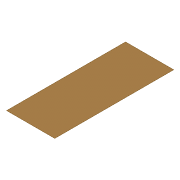
# Autodesk Inventor part: FE-00035-06
Saved by Autodesk Inventor 2012 (Build 160160000, 160)
## iProperties
Created: 2008-06-08
Part Number: FE-00035-06
Document SubType Name: Modeling
Designer: dfoster
Density: 1 g/cm^3
Description: Carpet, Playing Field
Material: Default
Title: Carpet, Playing Field
Author: dfoster
Autodesk Inventor part; units mm, degrees
ref_plane "YZ Plane" through (0, 0, 0) normal (1, 0, 0) x (0, 1, 0)
ref_plane "XZ Plane" through (0, 0, 0) normal (0, 1, 0) x (-1, 0, 0)
ref_plane "XY Plane" through (0, 0, 0) normal (0, 0, 1) x (1, 0, 0)
sketch "Sketch2" plane through (0, 0, 0) normal (0, 1, 0) x (-1, 0, 0)
  line L0 (4572, 11277.6) -> (-4572, 11277.6)
  line L1 (-4572, 11277.6) -> (-4572, -11277.6)
  line L2 (-4572, -11277.6) -> (4572, -11277.6)
  line L3 (4572, -11277.6) -> (4572, 11277.6)
  line L4 (0, -15788.64) -> (0, 15788.64) projected
  line L5 (-6400.8, 0) -> (6400.8, 0) projected
  dimension "d0" = 22555.2
  dimension "d1" = 9144
  dimension "d4" = 11277.6
  dimension "d5" = 4572
  constraints: 8 end point, 2 parallel, 1 horizontal, 1 perpendicular
  measures "d0" distance of L2.end L0.start
  measures "d1" distance of L1.end L2.end
  measures "d4" distance between parallel lines of L5 L2
  measures "d5" distance between parallel lines of L4 L1
extrude "Extrusion1" add sketch "Sketch2" along normal blind 6.35
equation "\"d4\" = 0.5 * d0"
equation "\"d5\" = 0.5 * d1"
body "Solid1"
